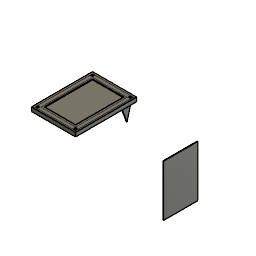
Ramecek Foto 10x15 (Autodesk Fusion 360 design; units mm, degrees)
Autodesk Fusion 360 part; units mm, degrees
sketch "Sketch1" plane through (0, 0, 0) normal (0, 1, 0) x (1, 0, 0)
  line L0 (60, 85) -> (-60, -85) construction
  line L1 (-60, 85) -> (60, -85) construction
  line L2 (49, 74) -> (-49, 74)
  line L3 (-49, 74) -> (-49, -74)
  line L4 (-49, -74) -> (49, -74)
  line L5 (49, -74) -> (49, 74)
  line L6 (49, 74) -> (-49, -74) construction
  line L7 (-49, 74) -> (49, -74) construction
  line L8 (-51, 76) -> (-51, -76)
  line L9 (-51, -76) -> (51, -76)
  line L10 (51, -76) -> (51, 76)
  line L11 (51, 76) -> (-51, 76)
  line L12 (-60, 85) -> (-60, -85)
  line L13 (-60, -85) -> (60, -85)
  line L14 (60, -85) -> (60, 85)
  line L15 (60, 85) -> (-60, 85)
  dimension "d10" = 98
  dimension "d11" = 148
  dimension "d19" = 2
  dimension "d20" = 9
  constraint coincident L0 origin
  constraint coincident L1 origin
  constraint horizontal L2
  constraint perpendicular L2 L3
  constraint parallel L2 L4
  constraint parallel L3 L5
  constraint coincident L6 origin
  constraint coincident L7 origin
  measures "d10" distance of L3.end L4.end
  measures "d11" distance of L2.end L3.end
extrude "Extrude1" add sketch "Sketch1" along normal blind 10 contours L12 L13 L14 L15 makes body 1
extrude "Extrude2" add sketch "Sketch1" along normal blind 7.5 contours L8 L9 L10 L11 bodies 1
sketch "Sketch3" plane through (0, 0, 0) normal (0, 1, 0) x (1, 0, 0)
  line L0 (136.909, 72.3092) -> (228.909, 72.3092)
  line L1 (228.909, 72.3092) -> (228.909, -69.6908)
  line L2 (228.909, -69.6908) -> (136.909, -69.6908)
  line L3 (136.909, -69.6908) -> (136.909, 72.3092)
  line L4 (242.959, 86.3592) -> (242.959, -83.7408)
  line L5 (242.959, -83.7408) -> (122.859, -83.7408)
  line L6 (122.859, -83.7408) -> (122.859, 86.3592)
  line L7 (122.859, 86.3592) -> (242.959, 86.3592)
  line L8 (247.959, -88.7408) -> (117.859, -88.7408)
  line L9 (117.859, -88.7408) -> (117.859, 91.3592)
  line L10 (117.859, 91.3592) -> (247.959, 91.3592)
  line L11 (247.959, 91.3592) -> (247.959, -88.7408)
  dimension "d16" = 92
  dimension "d17" = 142
  dimension "d18" = -14.05
  dimension "d21" = -5
  constraint horizontal L0
  constraint vertical L1
  constraint horizontal L2
  constraint vertical L3
  measures "d16" distance of L0.start L0.end
  measures "d17" distance of L0.start L2.end
extrude "Extrude3" add sketch "Sketch3" along normal blind 12 separate body contours L8 L9 L10 L11 makes body 2
extrude "Extrude4" add sketch "Sketch3" along normal blind 2 contours L4 L5 L6 L7 bodies 2
sketch "Sketch4" plane through (0, 10, 0) normal (0, 1, 0) x (-1, 0, 0)
  line L0 (51, -76) -> (-51, -76)
  line L1 (-51, -76) -> (-51, 76)
  line L2 (-51, 76) -> (51, 76)
  line L3 (51, 76) -> (51, -76)
  line L4 (-60, -85) -> (60, -85)
  line L5 (60, -85) -> (60, 85)
  line L6 (60, 85) -> (-60, 85)
  line L7 (-60, 85) -> (-60, -85)
  line L8 (53.15, -83.25) -> (58.25, -83.25)
  line L9 (58.25, -83.25) -> (58.25, -78.15)
  line L10 (58.25, -78.15) -> (53.15, -78.15)
  line L11 (53.15, -78.15) -> (53.15, -83.25)
  line L12 (53.15, -83.25) -> (58.25, -78.15) construction
  line L13 (58.25, -83.25) -> (53.15, -78.15) construction
  line L14 (0, -91.5702) -> (0, -78.4298)
  line L15 (68.3817, 0) -> (51.6183, 0)
  line L16 (-53.15, -78.15) -> (-53.15, -83.25)
  line L17 (-53.15, -83.25) -> (-58.25, -83.25)
  line L18 (-58.25, -83.25) -> (-58.25, -78.15)
  line L19 (-58.25, -78.15) -> (-53.15, -78.15)
  line L20 (53.15, 83.25) -> (58.25, 83.25)
  line L21 (58.25, 83.25) -> (58.25, 78.15)
  line L22 (58.25, 78.15) -> (53.15, 78.15)
  line L23 (53.15, 78.15) -> (53.15, 83.25)
  line L24 (-53.15, 78.15) -> (-53.15, 83.25)
  line L25 (-53.15, 83.25) -> (-58.25, 83.25)
  line L26 (-58.25, 83.25) -> (-58.25, 78.15)
  line L27 (-58.25, 78.15) -> (-53.15, 78.15)
  point P0 (55.7, -80.7)
  dimension "d27" = 5.1
  dimension "d83" = 1.75
  dimension "d84" = 1.75
  constraint horizontal L8
  constraint perpendicular L8 L9
  constraint parallel L8 L10
  constraint parallel L9 L11
  constraint coincident L12 P0
  constraint coincident L13 P0
  constraint perpendicular L0 L14
  constraint midpoint L4 L14
  constraint perpendicular L3 L15
  constraint midpoint L5 L15
  constraint equal L8 L9
  constraint symmetric L8.start L14 L16.end
  constraint symmetric L8.end L14 L17.end
  constraint symmetric L9.end L14 L18.end
  constraint symmetric L10.end L14 L16.start
  constraint symmetric L8.start L15 L20.start
  constraint symmetric L8.end L15 L20.end
  constraint symmetric L9.end L15 L21.end
  constraint symmetric L10.end L15 L22.end
  constraint symmetric L15 L16.start L24.start
  constraint symmetric L15 L16.end L24.end
  constraint symmetric L15 L17.end L25.end
  constraint symmetric L15 L18.end L26.end
  measures "d27" distance of L9 L11
  measures "d83" distance of L5 L9
  measures "d84" distance of L4 L8
copy_body "Body->Comp1" bodies 1 removing the originals makes body 3 in component "Spodní část rámečku"
copy_body "Body->Comp2" bodies 2 removing the originals makes body 4 in component "Horní část rámečku"
extrude "Extrude1'" cut sketch "Sketch4" against normal blind 1.9 contours L8 L9 L10 L11 | L16 L17 L18 L19 | L20 L21 L22 L23 | L24 L25 L26 L27 bodies 3 in component "Spodní část rámečku"
sketch "Sketch7" plane through (0, 0, 0) normal (0, 1, 0) x (1, 0, 0)
  line L0 (115.4319, 0.7999) -> (188.2572, 0.7999)
  line L1 (122.9878, 0.7999) -> (122.9878, 30.7999)
  line L2 (122.9878, 0.7999) -> (170.4622, 18.0792)
  line L3 (122.9878, 0.7999) -> (201, 0.7999) construction
  line L4 (122.9878, 30.7999) -> (170.4622, 18.0792)
  line L5 (122.9878, 30.7999) -> (117.9878, 30.7999)
  line L6 (117.9878, 30.7999) -> (117.9878, 0.7999)
  line L7 (117.9878, 0.7999) -> (122.9878, 0.7999)
  line L8 (122.9878, 0.7999) -> (122.9878, 30.7999)
  line L9 (122.9878, 30.7999) -> (185, 30.7999)
  dimension "d36" = 30
  dimension "d38" = 20
  dimension "d39" = 5
  dimension "d40" = 30
  dimension "d65" = 15
  constraint horizontal L0
  constraint coincident L0 L1.start
  constraint perpendicular L0 L1
  constraint horizontal L3
  constraint horizontal L5
  constraint vertical L6
  constraint horizontal L7
  constraint vertical L8
  constraint perpendicular L1 L9
  measures "d36" distance of L1.start L1.end
  measures "d38" angle of L2 L3
  measures "d39" distance of L1.end L5.end
  measures "d40" distance of L1.end L1.start
  measures "d65" angle of L4 L9
extrude "Extrude5" add sketch "Sketch7" along normal blind 2.4 separate body makes body 5
move_body "Move1" bodies 3 to x (-1, 0, 0) y (0, -1, 0) z (0, 0, 1) at (-120, 20, 0) in component "Spodní část rámečku"
move_body "Move1'" bodies 4 to x (1, 0, 0) y (0, 1, 0) z (0, 0, 1) at (42.7114, 0, -13.3808) in component "Horní část rámečku"
sketch "Sketch9" plane through (0, 20, 0) normal (0, 1, 0) x (-1, 0, 0)
  line L0 (169, 74) -> (169, -74)
  line L1 (169, -74) -> (71, -74)
  line L2 (71, -74) -> (71, 74)
  line L3 (71, 74) -> (169, 74)
  line L4 (60, -85) -> (180, -85)
  line L5 (180, -85) -> (180, 85)
  line L6 (180, 85) -> (60, 85)
  line L7 (60, 85) -> (60, -85)
  line L8 (64.2, -53.6) -> (66.8, -53.6)
  line L9 (66.8, -53.6) -> (66.8, -83.8)
  line L10 (66.8, -83.8) -> (64.2, -83.8)
  line L11 (64.2, -83.8) -> (64.2, -53.6)
  line L12 (60, -53.6) -> (71, -53.6)
  line L13 (65.5, -51.6305) -> (65.5, -55.5695)
  line L14 (120, 85) -> (120, 63)
  line L15 (175.8, -83.8) -> (175.8, -53.6)
  line L16 (175.8, -53.6) -> (173.2, -53.6)
  line L17 (173.2, -53.6) -> (173.2, -83.8)
  line L18 (173.2, -83.8) -> (175.8, -83.8)
  line L19 (61.2, 80.8) -> (91.4, 80.8)
  line L20 (91.4, 80.8) -> (91.4, 78.2)
  line L21 (91.4, 78.2) -> (61.2, 78.2)
  line L22 (61.2, 78.2) -> (61.2, 80.8)
  line L23 (87.6485, 79.5) -> (95.1515, 79.5)
  line L24 (51, 0) -> (91, 0)
  line L25 (61.2, -80.8) -> (91.4, -80.8)
  line L26 (91.4, -80.8) -> (91.4, -78.2)
  line L27 (91.4, -78.2) -> (61.2, -78.2)
  line L28 (61.2, -78.2) -> (61.2, -80.8)
  point P0 (120, 74)
  dimension "d44" = 2.6
  dimension "d45" = 30.2
  dimension "d46" = 1.2
  dimension "d55" = 30.2
  dimension "d56" = 2.6
  dimension "d57" = 1.2
  constraint horizontal L8
  constraint vertical L9
  constraint horizontal L10
  constraint vertical L11
  constraint coincident L7 L12.start
  constraint coincident L2 L12.end
  constraint perpendicular L2 L12
  constraint perpendicular L12 L13
  constraint midpoint L12 L13
  constraint midpoint L8 L12
  constraint perpendicular L3 L14
  constraint midpoint L3 L14
  constraint symmetric L8.start L14 L15.end
  constraint symmetric L8.end L14 L16.end
  constraint symmetric L9.end L14 L17.end
  constraint symmetric L10.end L14 L15.start
  constraint horizontal L19
  constraint vertical L20
  constraint horizontal L21
  constraint vertical L22
  constraint coincident L6 L14.start
  constraint midpoint L14 P0
  constraint perpendicular L14 L23
  constraint symmetric L14.start P0 L23
  constraint midpoint L20 L23
  constraint horizontal L24
  constraint midpoint L2 L24
  constraint symmetric L19.start L24 L25.start
  constraint symmetric L19.end L24 L25.end
  constraint symmetric L20.end L24 L26.end
  constraint symmetric L21.end L24 L27.end
  measures "d44" distance of L8.start L8.end
  measures "d45" distance of L8.start L10.end
  measures "d46" distance of L4 L10
  measures "d55" distance of L19.start L19.end
  measures "d56" distance of L19.start L21.end
  measures "d57" distance of L7 L22
extrude "Extrude2'" cut sketch "Sketch9" against normal blind 5.1 contours L8 L9 L11 L12 L27 | L9 L25 L26 L27 | L9 L11 L25 L27 | L9 L10 L11 L25 | L11 L25 L27 L28 | L15 L16 L17 L18 | L19 L20 L21 L22 bodies 3 in component "Spodní část rámečku"
sketch "Sketch10" plane through (0, 0, 0) normal (0, 1, 0) x (1, 0, 0)
  line L0 (167.5841, -53.6023) -> (319.0841, -53.6023)
  line L1 (319.0841, -53.6023) -> (319.0841, -155.1023)
  line L2 (319.0841, -155.1023) -> (167.5841, -155.1023)
  line L3 (167.5841, -155.1023) -> (167.5841, -53.6023)
  dimension "d50" = 151.5
  dimension "d51" = 101.5
  constraint horizontal L0
  constraint vertical L1
  constraint horizontal L2
  constraint vertical L3
  measures "d50" distance of L0.start L0.end
  measures "d51" distance of L0.start L2.end
extrude "Extrude6" add sketch "Sketch10" along normal blind 1.6 separate body makes body 6
copy_body "CopyPasteBodies1" bodies 6 makes body 7
move_body "Move1''" bodies 7 to x (0, -1, 0) y (1, 0, 0) z (0, 0, 1) at (317.4841, 320.6841, 0)
move_body "Move2" bodies 7 to x (1, 0, 0) y (0, 1, 0) z (0, 0, 1) at (70, 0, 0)
sketch "Sketch11" plane through (197.909, 2, 43.7408) normal (0, 1, 0) x (1, 0, 0)
  line L0 (73.7114, -12.5692) -> (-18.2886, -12.5692)
  line L1 (-18.2886, -12.5692) -> (-18.2886, 129.4308)
  line L2 (-18.2886, 129.4308) -> (73.7114, 129.4308)
  line L3 (73.7114, 129.4308) -> (73.7114, -12.5692)
  line L4 (-32.3386, 143.4808) -> (-32.3386, -26.6192)
  line L5 (-32.3386, -26.6192) -> (87.7614, -26.6192)
  line L6 (87.7614, -26.6192) -> (87.7614, 143.4808)
  line L7 (87.7614, 143.4808) -> (-32.3386, 143.4808)
  line L8 (-25.3386, -19.6192) -> (-30.5386, -19.6192)
  line L9 (-30.5386, -19.6192) -> (-30.5386, -24.8192)
  line L10 (-30.5386, -24.8192) -> (-25.3386, -24.8192)
  line L11 (-25.3386, -24.8192) -> (-25.3386, -19.6192)
  line L12 (-25.3386, -19.6192) -> (-30.5386, -24.8192) construction
  line L13 (-30.5386, -19.6192) -> (-25.3386, -24.8192) construction
  line L14 (27.7114, -3.4623) -> (27.7114, -21.6762)
  line L15 (-40.1147, 58.4308) -> (3.5375, 58.4308)
  line L16 (80.7614, -19.6192) -> (85.9614, -19.6192)
  line L17 (85.9614, -19.6192) -> (85.9614, -24.8192)
  line L18 (85.9614, -24.8192) -> (80.7614, -24.8192)
  line L19 (80.7614, -24.8192) -> (80.7614, -19.6192)
  line L20 (-25.3386, 136.4808) -> (-30.5386, 136.4808)
  line L21 (-30.5386, 136.4808) -> (-30.5386, 141.6808)
  line L22 (-30.5386, 141.6808) -> (-25.3386, 141.6808)
  line L23 (-25.3386, 141.6808) -> (-25.3386, 136.4808)
  line L24 (80.7614, 141.6808) -> (80.7614, 136.4808)
  line L25 (80.7614, 136.4808) -> (85.9614, 136.4808)
  line L26 (85.9614, 136.4808) -> (85.9614, 141.6808)
  line L27 (85.9614, 141.6808) -> (80.7614, 141.6808)
  point P0 (-27.9386, -22.2192)
  dimension "d58" = 5.2
  dimension "d59" = 5.2
  dimension "d61" = 1.8
  dimension "d62" = 1.8
  constraint horizontal L8
  constraint perpendicular L8 L9
  constraint parallel L8 L10
  constraint parallel L9 L11
  constraint coincident L12 P0
  constraint coincident L13 P0
  constraint perpendicular L0 L14
  constraint midpoint L0 L14
  constraint horizontal L15
  constraint midpoint L1 L15
  constraint symmetric L8.start L14 L16.start
  constraint symmetric L8.end L14 L16.end
  constraint symmetric L9.end L14 L17.end
  constraint symmetric L10.end L14 L18.end
  constraint symmetric L8.start L15 L20.start
  constraint symmetric L8.end L15 L20.end
  constraint symmetric L9.end L15 L21.end
  constraint symmetric L10.end L15 L22.end
  constraint symmetric L15 L16.start L24.end
  constraint symmetric L15 L16.end L25.end
  constraint symmetric L15 L17.end L26.end
  constraint symmetric L15 L18.end L24.start
  measures "d58" distance of L9.end L10.end
  measures "d59" distance of L8.end L9.end
  measures "d61" distance of L5 L10
  measures "d62" distance of L4 L9
extrude "Extrude2''" cut sketch "Sketch11" against normal blind 5 contours L8 L9 L10 L11 | L16 L17 L18 L19 | L20 L21 L22 L23 | L24 L25 L26 L27 bodies 4 in component "Horní část rámečku"
move_body "Move2'" bodies 3 to x (-1, 0, 0) y (0, -1, 0) z (0, 0, 1) at (-120, 40, 0) in component "Spodní část rámečku"
copy_body "Body->Comp3" bodies 5 removing the originals makes body 8 in component "Noha rámečku"
copy_body "Body->Comp4" bodies 6 removing the originals makes body 9 in component "Deska horizontálně"
component "Spodní část rámečku" placed x (1, 0, 0) y (0, 1, 0) z (0, 0, 1) at (0, 0, 0)
component "Horní část rámečku" placed x (-1, 0, 0) y (0, -1, 0) z (0, 0, 1) at (225.6204, 32.1, 14.69)
component "Noha rámečku" placed x (0, -1, 0) y (1, 0, 0) z (0, 0, 1) at (-55.7, 143.0878, -53.0001)
component "Deska horizontálně" placed x (0, 0, 1) y (0, 1, 0) z (-1, 0, 0) at (104.4023, 27.5, -243.3841)
component "Noha rámečku" placed x (0, -1, 0) y (1, 0, 0) z (0, 0, 1) at (53.3, 143.0878, -52.9001)
equation "foto_sirka = 100 mm"
equation "vule = 2 mm"
equation "foto_vyska = 150 mm"
equation "ram_sirka = 9 mm"
equation "ram_hloubka = 10 mm"
equation "d10 = foto_sirka - vule"
equation "d11 = foto_vyska - vule"
equation "d16 = foto_sirka - spadavka"
equation "d17 = foto_vyska - spadavka"
equation "d18 = -( ram_sirka + vule / 2 + spadavka / 2 + 0.05 mm )"
equation "d19 = vule"
equation "d20 = ram_sirka"
equation "d22 = ram_hloubka + vule"
equation "d24 = vule"
equation "dira = 5.1 mm"
equation "d27 = dira"
equation "d34 = -4.1 mm + 2.2 mm"
equation "spadavka = 8 mm"
equation "d50 = foto_vyska + 1.5 mm"
equation "d51 = foto_sirka + 1.5 mm"
named bodies: "Noha rámečku", "Deska horizontálně", "Deska vertikálně"
